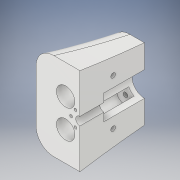
# Autodesk Inventor part: AA034
Saved by Autodesk Inventor 2017 SP1 (Build 210196100, 196)
## iProperties
Created: 2017-09-29
Part Number: AA034
Material: ABS Plastic
Document SubType Name: Modeling
Designer: Zach
Density: 1.06 g/cm^3
Appearance: CR White
Author: Zach
Autodesk Inventor part; units mm, degrees
ref_plane "YZ Plane" through (0, 0, 0) normal (1, 0, 0) x (0, 1, 0)
ref_plane "XZ Plane" through (0, 0, 0) normal (0, 1, 0) x (-1, 0, 0)
ref_plane "XY Plane" through (0, 0, 0) normal (0, 0, 1) x (1, 0, 0)
sketch "Sketch1" plane through (0, 0, 0) normal (0, 0, 1) x (1, 0, 0)
  line L0 (0, 0) -> (70, 0)
  line L1 (70, 0) -> (70, 77.5)
  line L2 (70, 77.5) -> (0, 77.5)
  line L3 (0, 77.5) -> (0, 0)
  dimension "d0" = 70
  dimension "d1" = 77.5
  constraints: 8 end point, 2 parallel, 1 horizontal, 1 perpendicular
  measures "d0" distance of L2.end L1.end
  measures "d1" distance of L1.end L0.end
extrude "Extrusion1" add sketch "Sketch1" along normal blind 70
sketch "Sketch3" plane through (0, 0, 70) normal (0, 0, 1) x (1, 0, 0)
  line L0 (0, 0) -> (70, 0) projected
  line L1 (70, 77.5) -> (0, 77.5) projected
  line L2 (70, 0) -> (35, 0)
  line L3 (35, 0) -> (35, 77.5)
  line L4 (35, 77.5) -> (70, 77.5)
  line L5 (70, 77.5) -> (70, 0)
  constraints: 8 end point, 2 parallel, 1 horizontal, 1 midpoint, 1 perpendicular
extrude "Extrusion3" cut sketch "Sketch3" against normal through all
sketch "Sketch4" plane through (0, 77.5, 70) normal (0, 1, 0) x (1, 0, 0)
  line L0 (0, 70) -> (0, 0) projected
  line L1 (0, 0) -> (-12.5, 0)
  line L2 (35, 70) -> (0, 70) projected
  arc A0 (-12.5, 0) -> (0, 70) centre (-1137.8005, 237.0626) ccw
  line L3 (-12.5, -10) -> (35, -10) construction
  dimension "d9" = 1150
  dimension "d54" = 47.5
  dimension "d55" = 10
  constraints: 4 end point, 2 horizontal, 2 point on circle, 2 vertical alignment, 1 centre point
  measures "d9" radius of A0
  measures "d54" distance of L3.start L3.end
  measures "d55" distance between parallel lines of L1 L3
extrude "Extrusion4" add sketch "Sketch4" against normal blind 77.5
sketch "Sketch5" plane through (35, 0, 70) normal (1, 0, 0) x (0, 0, -1)
  line L0 (0, 77.5) -> (0, 86.25)
  line L1 (0, 0) -> (0, -8.75)
  line L2 (0, 0) -> (0, 77.5) projected
  line L3 (70, 77.5) -> (70, 0) projected
  arc A0 (0, 86.25) -> (70, 77.5) centre (177.5728, 1222.4577) ccw
  arc A1 (70, 0) -> (0, -8.75) centre (177.5728, -1144.9577) ccw
  line L4 (0, 77.5) -> (70, 77.5) projected
  line L5 (70, 0) -> (0, 0) projected
  line L6 (-10, 86.25) -> (-10, -8.75) construction
  point P0 (-10, 38.75)
  point P1 (0, 38.75)
  dimension "d14" = 1150
  dimension "d15" = 1150
  dimension "d52" = 10
  dimension "d53" = 95
  constraints: 6 end point, 4 point on circle, 3 horizontal alignment, 3 vertical, 2 centre point, 2 midpoint
  measures "d14" radius of A0
  measures "d15" radius of A1
  measures "d52" distance between parallel lines of L2 L6
  measures "d53" distance of L6.start L6.end
extrude "Extrusion5" add sketch "Sketch5" against normal blind 55 contours L0 A0 L4 | L5 A1 L1
sketch "Sketch6" plane through (-20, 0, 0) normal (0, 1, 0) x (1, 0, 0)
  line L0 (20, 0) -> (0, 0) projected
  line L1 (0, -70) -> (0, 0) projected
  arc A0 (7.5, -70) -> (20, 0) centre (-1117.8005, 167.0626) ccw projected
  line L2 (7.5, -70) -> (0, -70) projected
extrude "Extrusion6" cut sketch "Sketch6" along normal through all both and the other way through all
fillet "Fillet3" radius 19.35 2 edges at (-5.7463, 81.368, 35.3063) (-5.7463, -3.868, 35.3063)
ref_plane "Work Plane3" through (0, 0, 65) normal (0, 0, 1) x (1, 0, 0)
sketch "Sketch24" plane through (0, 0, 65) normal (0, 0, 1) x (1, 0, 0)
  line L0 (35, 77.5) -> (35, 0) projected
  circle A0 centre (35, 38.75) radius 11.5
  point P0 (0, 0)
  dimension "d85" = 23
  constraints: 1 centre point, 1 midpoint
  measures "d85" diameter of A0
extrude "Extrusion20" cut sketch "Sketch24" against normal blind 9
sketch "Sketch26" plane through (0, 0, 70) normal (0, 0, 1) x (1, 0, 0)
  line L0 (35, 77.5) -> (35, 0) projected
  circle A0 centre (35, 38.75) radius 4.5
  point P0 (0, 0)
  dimension "d88" = 9
  constraints: 1 centre point, 1 midpoint
  measures "d88" diameter of A0
extrude "Extrusion21" cut sketch "Sketch26" against normal blind 50
ref_plane "Work Plane4" through (0, 0, 35) normal (0, 0, 1) x (1, 0, 0)
sketch "Sketch28" plane through (0, 0, 35) normal (0, 0, 1) x (1, 0, 0)
  line L0 (35, 43.25) -> (35, 34.25) projected
  circle A0 centre (35, 38.75) radius 11.5
  point P0 (0, 0)
  dimension "d92" = 23
  constraints: 1 centre point, 1 midpoint
  measures "d92" diameter of A0
extrude "Extrusion22" cut sketch "Sketch28" along normal blind 9
sketch "Sketch29" plane through (0, 0, 35) normal (0, 0, 1) x (1, 0, 0)
  line L0 (35, 43.25) -> (35, 34.25)
  circle A0 centre (35, 38.75) radius 11.5
  point P0 (0, 0)
  dimension "d96" = 23
  constraints: 2 end point, 1 centre point, 1 midpoint
  measures "d96" diameter of A0
extrude "Extrusion23" cut sketch "Sketch29" against normal through all
sketch "Sketch32" plane through (0, 0, 70) normal (0, 0, 1) x (1, 0, 0)
  circle A0 centre (19.5, 23.25) radius 2.5
  circle A1 centre (19.5, 54.25) radius 2.5
  line L0 (19.5, 54.25) -> (19.5, 23.25) construction
  arc A2 (35, 43.25) -> (35, 34.25) centre (35, 38.75) ccw projected
  line L1 (35, 86.25) -> (35, 43.25) projected
  point P0 (0, 0)
  point P1 (19.5, 38.75)
  dimension "d105" = 5
  dimension "d106" = 5
  dimension "d107" = 15.5
  dimension "d108" = 31
  constraints: 2 centre point, 2 end point, 1 horizontal alignment, 1 midpoint, 1 vertical
  measures "d105" diameter of A0
  measures "d106" diameter of A1
  measures "d107" distance between parallel lines of L1 L0
  measures "d108" distance of L0.start L0.end
extrude "Extrusion26" cut sketch "Sketch32" against normal through all
sketch "Sketch33" plane through (0, 0, 70) normal (0, 0, 1) x (1, 0, 0)
  circle A0 centre (19.5, 54.25) radius 2.5 projected
  circle A1 centre (19.5, 23.25) radius 2.5 projected
  circle A2 centre (19.5, 54.25) radius 10
  circle A3 centre (19.5, 23.25) radius 10
  point P0 (0, 0)
  dimension "d111" = 20
  dimension "d112" = 20
  constraints: 2 centre point, 2 coincident
  measures "d111" diameter of A2
  measures "d112" diameter of A3
extrude "Extrusion27" cut sketch "Sketch33" against normal blind 65
sketch "Sketch34" plane through (35, 50.25, 65) normal (1, 0, 0) x (0, 0, -1)
  circle A0 centre (31, 13.5) radius 2.5
  circle A1 centre (31, -36.5) radius 2.5
  line L0 (31, -36.5) -> (31, 13.5) construction
  line L1 (-5, -16) -> (-5, -7) projected
  line L2 (21, -7) -> (21, 0) projected
  point P0 (65, -50.25)
  point P1 (31, -11.5)
  point P2 (-5, -11.5)
  dimension "d115" = 5
  dimension "d116" = 5
  dimension "d117" = 50
  dimension "d118" = 10
  constraints: 2 centre point, 2 end point, 2 midpoint, 1 horizontal alignment
  measures "d115" diameter of A0
  measures "d116" diameter of A1
  measures "d117" distance of L0.start L0.end
  measures "d118" distance between parallel lines of L2 L0
extrude "Extrusion28" cut sketch "Sketch34" against normal through all
sketch "Sketch36" plane through (0, 0, 44) normal (0, 0, -1) x (-1, 0, 0)
  arc A0 (-35, 34.25) -> (-35, 43.25) centre (-35, 38.75) ccw projected
  circle A1 centre (-35, 38.75) radius 13.5
  point P0 (0, 0)
  dimension "d125" = 27
  constraints: 1 centre point, 1 coincident
  measures "d125" diameter of A1
extrude "Extrusion30" cut sketch "Sketch36" along normal through all
sketch "Sketch38" plane through (0, 0, 65) normal (0, 0, 1) x (1, 0, 0)
  arc A0 (35, 43.25) -> (35, 34.25) centre (35, 38.75) ccw projected
  line L0 (35, 27.25) -> (35, 34.25) projected
  arc A1 (35, 50.25) -> (35, 27.25) centre (35, 38.75) ccw projected
  line L1 (35, 43.25) -> (35, 50.25) projected
  point P0 (0, 0)
extrude "Extrusion32" add sketch "Sketch38" against normal blind 9
sketch "Sketch37" plane through (0, 0, 44) normal (0, 0, -1) x (-1, 0, 0)
  circle A0 centre (-25.475, 38.75) radius 1.5
  arc A1 (-35, 34.25) -> (-35, 43.25) centre (-35, 38.75) ccw projected
  circle A2 centre (-30.2375, 46.9989) radius 1.5
  circle A3 centre (-39.7625, 46.9989) radius 1.5
  circle A4 centre (-44.525, 38.75) radius 1.5
  circle A5 centre (-39.7625, 30.5011) radius 1.5
  circle A6 centre (-30.2375, 30.5011) radius 1.5
  point P0 (0, 0)
  dimension "d128" = 3
  dimension "d129" = 9.525
  dimension "d132" = 360
  constraints: 6 centre point, 1 horizontal alignment, 13 other
  measures "d128" diameter of A0
  measures "d129" distance of A1.centre A0.centre
extrude "Extrusion31" cut sketch "Sketch37" against normal through all
body "Solid1"
